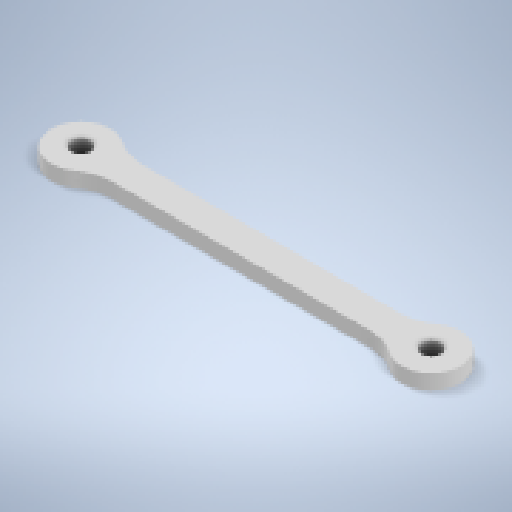
# Autodesk Inventor part: Рычаг
Saved by Autodesk Inventor 2023.2 (Build 272271030, 271C)
## iProperties
Created: 2024-02-06
Part Number: Рычаг
Material: Типовые
Document SubType Name: Modeling
Designer: I9232
Density: 1 g/cm^3
Appearance: По умолчанию
Author: I9232
Autodesk Inventor part; units mm, degrees
ref_plane "YZ Plane" through (0, 0, 0) normal (1, 0, 0) x (0, 1, 0)
ref_plane "XZ Plane" through (0, 0, 0) normal (0, 1, 0) x (-1, 0, 0)
ref_plane "XY Plane" through (0, 0, 0) normal (0, 0, 1) x (1, 0, 0)
sketch "Эскиз1" plane through (0, 0, 0) normal (0, 1, 0) x (-1, 0, 0)
  arc A0 (29.8038, -3) -> (29.8038, 3) centre (35, 0) ccw
  line L0 (30.0057, 0) -> (28.0258, 0)
  circle A1 centre (35, 0) radius 1.9
  arc A2 (-29.8038, 3) -> (-29.8038, -3) centre (-35, 0) ccw
  line L1 (-29.8038, -3) -> (29.8038, -3)
  line L2 (-29.8038, 3) -> (29.8038, 3)
  circle A3 centre (-35, 0) radius 1.9
  line L3 (32.9518, 0) -> (37.6343, 0) construction
  line L4 (14.11, -3) -> (14.11, 3)
  line L5 (0, -3) -> (0, 3)
  point P0 (0, 0)
  point P1 (25.2378, -3)
  point P2 (25.2378, 3)
  point P3 (0, 0)
  dimension "d2" = 6
  dimension "d3" = 35
  dimension "d4" = 3.8
  dimension "d9" = 6
  constraints: 12 end point, 5 point on line, 4 centre point, 4 point on circle, 3 coincident, 3 midpoint, 2 equal radius, 2 horizontal, 2 symmetric about line, 1 perpendicular
  measures "d2" radius of A0
  measures "d3" distance of point (0, 0) A0.centre
  measures "d4" diameter of A1
  measures "d9" distance between parallel lines of L2 L1
extrude "Выдавливание1" add sketch "Эскиз1" along normal mid plane 3
fillet "Сопряжение1" radius 10 4 edges at (-29.8038, 0, 3) (-29.8038, 0, -3) (29.8038, 0, -3) (29.8038, 0, 3)
